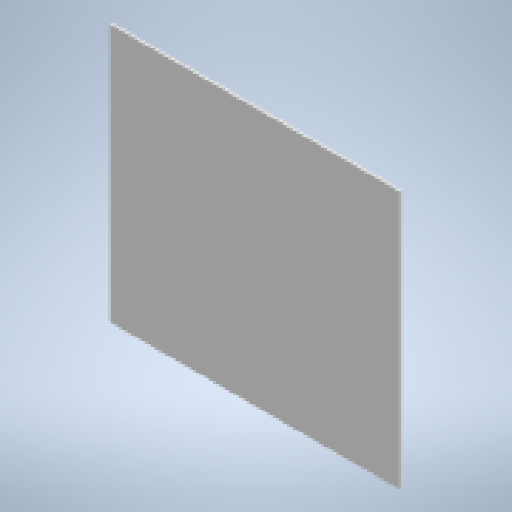
# Autodesk Inventor part: Floor
Saved by Autodesk Inventor 2025.2 (Build 292293000, 293)
## iProperties
Created: 2025-04-23
Part Number: Floor
Material: Generic
Document SubType Name: Modeling
Designer: powel
Density: 1 g/cm^3
Appearance: Default
Author: powel
Autodesk Inventor part; units mm, degrees
ref_plane "YZ Plane" through (0, 0, 0) normal (1, 0, 0) x (0, 1, 0)
ref_plane "XZ Plane" through (0, 0, 0) normal (0, 1, 0) x (-1, 0, 0)
ref_plane "XY Plane" through (0, 0, 0) normal (0, 0, 1) x (1, 0, 0)
sketch "Sketch1" plane through (0, 0, 0) normal (0, 0, 1) x (1, 0, 0)
  line L0 (0, 0) -> (-288, 0)
  line L1 (-288, 0) -> (-288, -256)
  line L2 (-288, -256) -> (0, -256)
  line L3 (0, -256) -> (0, 0)
  dimension "d0" = 288
  dimension "d1" = 256
  constraints: 8 end point, 2 parallel, 1 horizontal, 1 perpendicular
  measures "d0" distance of L2.end L1.end
  measures "d1" distance of L1.end L0.end
extrude "Extrusion1" add sketch "Sketch1" along normal blind 2.54
body "Solid1"
